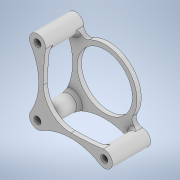
# Autodesk Inventor part: TopMotorMount
Saved by Autodesk Inventor 2020 (Build 240168000, 168)
## iProperties
Created: 2019-04-28
Part Number: TopMotorMount
Material: Generic
Document SubType Name: Modeling
Designer: Connor
Density: 1 g/cm^3
Appearance: Default
Author: Connor
Autodesk Inventor part; units mm, degrees
ref_plane "YZ Plane" through (0, 0, 0) normal (1, 0, 0) x (0, 1, 0)
ref_plane "XZ Plane" through (0, 0, 0) normal (0, 1, 0) x (-1, 0, 0)
sketch "Sketch1" plane through (0, 0, 0) normal (0, 0, 1) x (1, 0, 0)
  circle A0 centre (0, 0) radius 2.5
  circle A1 centre (47.14, 0) radius 2.5
  circle A2 centre (0, 47.14) radius 2.5
  line L0 (0, 47.14) -> (0, 0) construction
  line L1 (0, 0) -> (47.14, 0) construction
  circle A3 centre (0, 0) radius 5.7
  circle A4 centre (0, 47.14) radius 5.7
  circle A5 centre (47.14, 0) radius 5.7
  line L2 (0, 47.14) -> (47.14, 0) construction
  line L3 (0, 0) -> (23.57, 23.57) construction
  circle A6 centre (23.57, 23.57) radius 19.5
  circle A7 centre (23.57, 23.57) radius 22.7
  arc A8 (5.7, 47.14) -> (12.326772, 43.290036) centre (10.131745, 47.14) ccw
  arc A9 (43.290036, 12.326772) -> (47.14, 5.7) centre (47.14, 10.131745) ccw
  arc A10 (44.191416, -4.8781) -> (2.948584, -4.8781) centre (23.57, -38.993912) ccw
  arc A11 (-4.8781, 2.948584) -> (-4.8781, 44.191416) centre (-38.993912, 23.57) ccw
  dimension "d0" = 5
  dimension "d3" = 47.14
  dimension "d5" = 3.2
  dimension "d7" = 39
  dimension "d8" = 3.2
  constraints: 16 point on circle, 12 centre point, 10 tangent, 8 end point, 5 equal radius, 2 coincident, 2 perpendicular, 1 horizontal alignment, 1 midpoint, 1 vertical
  measures "d0" diameter of A0
  measures "d3" distance of L0.start L0.end
  measures "d5" radial gap between concentric circles of A0 A3
  measures "d7" diameter of A6
  measures "d8" radial gap between concentric circles of A6 A7
extrude "Extrusion1" add sketch "Sketch1" along normal blind 26.9
ref_plane "Work Plane1" through (0, 0, 23.9) normal (0, 0, 1) x (1, 0, 0)
sketch "Sketch3" plane through (0, 0, 23.9) normal (0, 0, 1) x (1, 0, 0)
  arc A0 (43.290036, 12.326772) -> (47.14, 5.7) centre (47.14, 10.131745) ccw
  arc A1 (43.290036, 12.326772) -> (12.326772, 43.290036) centre (23.57, 23.57) ccw
  arc A2 (5.7, 47.14) -> (12.326772, 43.290036) centre (10.131745, 47.14) ccw
  arc A3 (5.7, 47.14) -> (-4.8781, 44.191416) centre (0, 47.14) ccw
  arc A4 (-4.8781, 2.948584) -> (-4.8781, 44.191416) centre (-38.993912, 23.57) ccw
  arc A5 (-4.8781, 2.948584) -> (2.948584, -4.8781) centre (0, 0) ccw
  arc A6 (44.191416, -4.8781) -> (2.948584, -4.8781) centre (23.57, -38.993912) ccw
  arc A7 (44.191416, -4.8781) -> (47.14, 5.7) centre (47.14, 0) ccw
  circle A8 centre (47.14, 0) radius 2.5
  circle A9 centre (0, 0) radius 2.5
  circle A10 centre (23.57, 23.57) radius 19.5
  circle A11 centre (0, 47.14) radius 2.5
  arc A12 (5.7, 47.14) -> (12.326772, 43.290036) centre (10.131745, 47.14) ccw
  circle A13 centre (0, 47.14) radius 5.7
  circle A14 centre (0, 0) radius 5.7
  arc A15 (-4.8781, 2.948584) -> (-4.8781, 44.191416) centre (-38.993912, 23.57) ccw
  arc A16 (44.191416, -4.8781) -> (47.14, 5.7) centre (47.14, 0) ccw
  circle A17 centre (47.14, 0) radius 5.7
  point P0 (-4.8781, 44.191416)
  point P1 (-4.8781, 2.948584)
  point P2 (2.948584, -4.8781)
  point P3 (44.191416, -4.8781)
  constraints: 3 coincident, 1 centre point, 1 tangent, 6 other
extrude "Extrusion2" cut sketch "Sketch3" against normal blind 20.9 contours A0 A17 A6 A14 A4 A13 A2 A1
sketch "Sketch4" plane through (0, 0, 26.9) normal (0, 0, 1) x (1, 0, 0)
  arc A0 (43.290036, 12.326772) -> (47.14, 5.7) centre (47.14, 10.131745) ccw
  arc A1 (43.290036, 12.326772) -> (12.326772, 43.290036) centre (23.57, 23.57) ccw
  arc A2 (5.7, 47.14) -> (12.326772, 43.290036) centre (10.131745, 47.14) ccw
  arc A3 (5.7, 47.14) -> (-4.8781, 44.191416) centre (0, 47.14) ccw
  arc A4 (-4.8781, 2.948584) -> (-4.8781, 44.191416) centre (-38.993912, 23.57) ccw
  arc A5 (-4.8781, 2.948584) -> (2.948584, -4.8781) centre (0, 0) ccw
  arc A6 (44.191416, -4.8781) -> (2.948584, -4.8781) centre (23.57, -38.993912) ccw
  arc A7 (44.191416, -4.8781) -> (47.14, 5.7) centre (47.14, 0) ccw
  circle A8 centre (47.14, 0) radius 2.5
  circle A9 centre (0, 0) radius 2.5
  circle A10 centre (23.57, 23.57) radius 19.5
  circle A11 centre (0, 47.14) radius 2.5
  arc A12 (5.7, 47.14) -> (-4.8781, 44.191416) centre (0, 47.14) ccw
  arc A13 (2.948584, -4.8781) -> (-4.8781, 2.948584) centre (0, 0) ccw
  arc A14 (5.645739, 46.355377) -> (5.645739, 0.784623) centre (169.597546, 23.57) ccw
  arc A15 (-4.8781, 44.191416) -> (5.7, 47.14) centre (0, 47.14) ccw
  circle A16 centre (23.57, 23.57) radius 19.5
  arc A17 (47.14, 5.7) -> (44.191416, -4.8781) centre (47.14, 0) ccw
  arc A18 (0.784623, 5.645739) -> (46.355377, 5.645739) centre (23.57, 169.597546) ccw
  point P0 (4.07, 23.57)
  point P1 (23.57, 4.07)
  constraints: 8 point on circle, 6 tangent, 2 centre point
extrude "Extrusion3" cut sketch "Sketch4" against normal up to surface (3 mm away) contours A0 A17 A18 A10 A14 A15 A2 A1
fillet "Fillet1" radius 2 6 edges at (1.5305, 41.6493, 3) (4.0305, 4.0305, 3) (41.6493, 1.5305, 3) (1.148, 41.5568, 23.9) (41.5568, 1.148, 23.9) (4.0305, 4.0305, 23.9)
body "Solid1"
